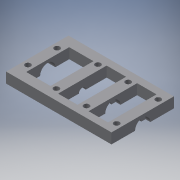
# Autodesk Inventor part: frame 1
Saved by Autodesk Inventor 2016 (Build 200138000, 138)
## iProperties
Created: 2017-06-14
Part Number: frame 1
Material: Generic
Document SubType Name: Modeling
Designer: RMcComber
Density: 1 g/cm^3
Appearance: Default
Author: RMcComber
Autodesk Inventor part; units mm, degrees
ref_plane "YZ Plane" through (0, 0, 0) normal (1, 0, 0) x (0, 1, 0)
ref_plane "XZ Plane" through (0, 0, 0) normal (0, 1, 0) x (-1, 0, 0)
ref_plane "XY Plane" through (0, 0, 0) normal (0, 0, 1) x (1, 0, 0)
sketch "Sketch1" plane through (0, 0, 0) normal (0, 0, 1) x (1, 0, 0)
  line L0 (51, -45) -> (-51, -45)
  line L1 (-51, -45) -> (-51, 45)
  line L2 (-51, 45) -> (51, 45)
  line L3 (51, 45) -> (51, -45)
  line L4 (51, -45) -> (-51, 45) construction
  line L5 (-51, -45) -> (51, 45) construction
  line L6 (-22, 0) -> (22, 0) construction
  line L7 (-36, 35) -> (-8, 35)
  line L8 (-8, 35) -> (-8, -35)
  line L9 (-8, -35) -> (-36, -35)
  line L10 (-36, -35) -> (-36, 35)
  line L11 (-36, 35) -> (-8, -35) construction
  line L12 (-8, 35) -> (-36, -35) construction
  line L13 (36, 35) -> (8, 35)
  line L14 (8, 35) -> (8, -35)
  line L15 (8, -35) -> (36, -35)
  line L16 (36, -35) -> (36, 35)
  line L17 (36, 35) -> (8, -35) construction
  line L18 (8, 35) -> (36, -35) construction
  point P0 (0, 0)
  point P1 (0, 0)
  dimension "d0" = 16
  dimension "d1" = 28
  dimension "d2" = 28
  dimension "d3" = 70
  dimension "d4" = 10
  dimension "d5" = 15
  constraints: 38 end point, 8 midpoint, 7 parallel, 4 perpendicular, 3 horizontal
  measures "d0" distance between parallel lines of L14 L8
  measures "d1" distance of L7.start L7.end
  measures "d2" distance of L13.start L13.end
  measures "d3" distance of L15.end L13.start
  measures "d4" distance between parallel lines of L7 L2
  measures "d5" distance between parallel lines of L1 L10
extrude "Extrusion1" add sketch "Sketch1" along normal blind 15
sketch "Sketch2" plane through (51, -45, 0) normal (1, 0, 0) x (0, 0, -1)
  circle A0 centre (0, 45) radius 5
  point P0 (0, 45)
  dimension "d8" = 10
  constraints: 1 centre point, 1 coincident
  measures "d8" diameter of A0
extrude "Extrusion2" cut sketch "Sketch2" against normal through all
sketch "Sketch3" plane through (51, -45, 15) normal (1, 0, 0) x (0, 0, -1)
  arc A0 (15, 50) -> (15, 40) centre (15, 45) ccw projected
  circle A1 centre (15, 45) radius 11
  dimension "d11" = 22
  constraints: 1 centre point, 1 coincident
  measures "d11" diameter of A1
extrude "Extrusion3" cut sketch "Sketch3" against normal blind 7
sketch "Sketch4" plane through (-51, -45, 15) normal (-1, 0, 0) x (0, 0, 1)
  arc A0 (-15, 40) -> (-15, 50) centre (-15, 45) ccw projected
  circle A1 centre (-15, 45) radius 11
  dimension "d14" = 22
  constraints: 1 centre point, 1 coincident
  measures "d14" diameter of A1
extrude "Extrusion4" cut sketch "Sketch4" against normal blind 7
sketch "Sketch5" plane through (-8, -35, 15) normal (-1, 0, 0) x (0, 0, 1)
  arc A0 (-15, 30) -> (-15, 40) centre (-15, 35) ccw projected
  circle A1 centre (-15, 35) radius 11
  dimension "d17" = 22
  constraints: 1 centre point, 1 coincident
  measures "d17" diameter of A1
extrude "Extrusion5" cut sketch "Sketch5" against normal blind 7
sketch "Sketch6" plane through (8, -35, 15) normal (1, 0, 0) x (0, 0, -1)
  arc A0 (15, 40) -> (15, 30) centre (15, 35) ccw projected
  circle A1 centre (15, 35) radius 11
  dimension "d20" = 22
  constraints: 1 centre point, 1 coincident
  measures "d20" diameter of A1
extrude "Extrusion6" cut sketch "Sketch6" against normal blind 7
sketch "Sketch7" plane through (0, 0, 15) normal (0, 0, 1) x (1, 0, 0)
  line L0 (-36, -35) -> (-36, 35) projected
  line L1 (-51, 45) -> (-51, -45) projected
  line L2 (0, 30) -> (0, -30) construction
  circle A0 centre (0, 30) radius 4
  circle A1 centre (0, -30) radius 4
  line L3 (43.5, -30) -> (-43.5, -30) construction
  line L4 (-43.5, -30) -> (-43.5, 30) construction
  line L5 (-43.5, 30) -> (43.5, 30) construction
  line L6 (43.5, 30) -> (43.5, -30) construction
  line L7 (43.5, -30) -> (-43.5, 30) construction
  line L8 (-43.5, -30) -> (43.5, 30) construction
  circle A2 centre (-43.5, 30) radius 4
  circle A3 centre (-43.5, -30) radius 4
  circle A4 centre (43.5, -30) radius 4
  circle A5 centre (43.5, 30) radius 4
  point P0 (0, 0)
  point P1 (0, 0)
  dimension "d23" = 60
  dimension "d24" = 8
  dimension "d25" = 7.5
  dimension "d26" = 87
  constraints: 14 end point, 7 coincident, 6 centre point, 5 equal radius, 4 midpoint, 3 parallel, 1 horizontal, 1 perpendicular
  measures "d23" distance of L2.start L2.end
  measures "d24" diameter of A0
  measures "d25" distance between parallel lines of L0 L4
  measures "d26" distance of L4.end L5.end
extrude "Extrusion7" cut sketch "Sketch7" against normal through all
sketch "Sketch8" plane through (0, 0, 15) normal (0, 0, 1) x (1, 0, 0)
  line L0 (-51, 45) -> (-86, 45)
  line L1 (-86, 45) -> (-86, 31)
  line L2 (-86, 31) -> (-51, 31)
  line L3 (-51, 31) -> (-51, 45)
  line L4 (-51, -45) -> (-86, -45)
  line L5 (-86, -45) -> (-86, -31)
  line L6 (-86, -31) -> (-51, -31)
  line L7 (-51, -31) -> (-51, -45)
  line L8 (-86, 45) -> (-101, 45)
  line L9 (-101, 45) -> (-101, -45)
  line L10 (-101, -45) -> (-86, -45)
  line L11 (-86, -45) -> (-86, 45)
  point P0 (0, 0)
  dimension "d29" = 14
  dimension "d30" = 15
  dimension "d31" = 35
  constraints: 24 end point, 6 parallel, 3 horizontal, 3 perpendicular, 1 collinear
  measures "d29" distance between parallel lines of L0 L2
  measures "d30" distance between parallel lines of L1 L9
  measures "d31" distance of L0.start L0.end
extrude "Extrusion8" add sketch "Sketch8" against normal up to surface (15 mm away)
sketch "Sketch9" plane through (-101, -45, 15) normal (-1, 0, 0) x (0, 0, 1)
  circle A0 centre (-15, 45) radius 11
  dimension "d34" = 22
  constraints: 1 centre point, 1 coincident
  measures "d34" diameter of A0
extrude "Extrusion9" cut sketch "Sketch9" against normal up to surface (50 mm away)
sketch "Sketch10" plane through (0, 0, 0) normal (0, 0, -1) x (-1, 0, 0)
  line L0 (101, -11) -> (86, -11) projected
  circle A0 centre (43.5, 30) radius 4 projected
  circle A1 centre (0, 30) radius 4 projected
  circle A2 centre (-43.5, 30) radius 4 projected
  line L1 (86, 11) -> (101, 11) projected
  line L2 (101, 11) -> (101, 45) projected
  line L3 (101, 45) -> (-51, 45) projected
  line L4 (-51, 45) -> (-51, 11) projected
  line L5 (-51, 11) -> (-44, 11) projected
  line L6 (-44, 11) -> (-44, 5) projected
  line L7 (-44, 5) -> (-36, 5) projected
  line L8 (-36, 5) -> (-36, 35) projected
  line L9 (-36, 35) -> (-8, 35) projected
  line L10 (-8, 35) -> (-8, 11) projected
  line L11 (-8, 11) -> (-1, 11) projected
  line L12 (-1, 11) -> (-1, 5) projected
  line L13 (-1, 5) -> (1, 5) projected
  line L14 (1, 5) -> (1, 11) projected
  line L15 (1, 11) -> (8, 11) projected
  line L16 (8, 11) -> (8, 35) projected
  line L17 (8, 35) -> (36, 35) projected
  line L18 (36, 35) -> (36, 5) projected
  line L19 (36, 5) -> (44, 5) projected
  line L20 (44, 5) -> (44, 11) projected
  line L21 (44, 11) -> (51, 11) projected
  line L22 (51, 11) -> (51, 31) projected
  line L23 (51, 31) -> (86, 31) projected
  line L24 (86, 31) -> (86, 11) projected
  line L25 (93.5, 11) -> (93.5, 21) construction
  line L26 (93.5, -11) -> (93.5, -21) construction
  circle A3 centre (93.5, 21) radius 4
  circle A4 centre (93.5, -21) radius 4
  point P0 (0, 0)
  dimension "d37" = 8
  dimension "d38" = 10
  constraints: 4 end point, 2 centre point, 2 coincident, 2 collinear, 2 midpoint, 1 equal radius, 1 parallel
  measures "d37" diameter of A3
  measures "d38" distance of L25.start L25.end
extrude "Extrusion10" cut sketch "Sketch10" against normal through all contours A3 | A4
body "Solid1"
